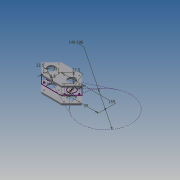
# Autodesk Inventor part: Part5
Saved by Autodesk Inventor 2013 (Build 170138000, 138)
## iProperties
Created: 2017-03-27
Part Number: Part5
Material: Generic
Document SubType Name: Modeling
Designer: employee
Density: 1 g/cm^3
Author: employee
Autodesk Inventor part; units mm, degrees
ref_plane "YZ Plane" through (0, 0, 0) normal (1, 0, 0) x (0, 1, 0)
ref_plane "XZ Plane" through (0, 0, 0) normal (0, 1, 0) x (-1, 0, 0)
ref_plane "XY Plane" through (0, 0, 0) normal (0, 0, 1) x (1, 0, 0)
sketch "Sketch1" plane through (0, 0, 0) normal (0, 0, 1) x (1, 0, 0)
  circle A0 centre (0, 0) radius 5.093 construction
  circle A1 centre (99, 0) radius 74.8028 construction
  line L0 (46.3283, 53.1146) -> (-3.5862, 3.6163) construction
  line L1 (-3.5862, -3.6163) -> (46.3283, -53.1146) construction
  circle A2 centre (-60, 0) radius 5.093 construction
  line L2 (66.2044, 67.2303) -> (-62.2329, 4.5774) construction
  line L3 (66.2044, -67.2303) -> (-62.2329, -4.5774) construction
  line L4 (-60, -29.6985) -> (-89.6985, 0) construction
  line L5 (-89.6985, 0) -> (-60, 29.6985) construction
  line L6 (-60, 29.6985) -> (-30.3015, 0) construction
  line L7 (-30.3015, 0) -> (-60, -29.6985) construction
  line L8 (-29.6985, 0) -> (0, 29.6985) construction
  line L9 (0, 29.6985) -> (29.6985, 0) construction
  line L10 (29.6985, 0) -> (0, -29.6985) construction
  line L11 (0, -29.6985) -> (-29.6985, 0) construction
  circle A3 centre (-60, 0) radius 11.25
  circle A4 centre (0, 0) radius 11.25
  line L12 (-21.9203, 0) -> (0, 21.9203) construction
  line L13 (0, 21.9203) -> (21.9203, 0) construction
  line L14 (21.9203, 0) -> (0, -21.9203) construction
  line L15 (0, -21.9203) -> (-21.9203, 0) construction
  line L16 (-60, 21.9203) -> (-38.0797, 0) construction
  line L17 (-38.0797, 0) -> (-60, -21.9203) construction
  line L18 (-60, -21.9203) -> (-81.9203, 0) construction
  line L19 (-81.9203, 0) -> (-60, 21.9203) construction
  circle A5 centre (-81.9203, 0) radius 1.75
  circle A6 centre (-60, 21.9203) radius 1.75
  circle A7 centre (-38.0797, 0) radius 1.75
  circle A8 centre (-60, -21.9203) radius 1.75
  circle A9 centre (0, -21.9203) radius 1.75
  circle A10 centre (-21.9203, 0) radius 1.75
  circle A11 centre (0, 21.9203) radius 1.75
  circle A12 centre (21.9203, 0) radius 1.75
  line L20 (-89.6985, 0) -> (-60, 29.6985)
  line L21 (-60, 29.6985) -> (0, 29.6985)
  line L22 (0, 29.6985) -> (29.6985, 0)
  line L23 (29.6985, 0) -> (0, -29.6985)
  line L24 (0, -29.6985) -> (-60, -29.6985)
  line L25 (-60, -29.6985) -> (-89.6985, 0)
  line L26 (-9.9329, 18.9203) -> (10.7782, 18.9203)
  dimension "d0" = 10.1859
  dimension "d2" = 149.6056
  dimension "d3" = 99
  dimension "d6" = 159
  dimension "d7" = 42
  dimension "d8" = 22.5
  dimension "d9" = 22.5
  dimension "d10" = 31
  dimension "d11" = 3.5
  dimension "d17" = 3
  constraints: 54 end point, 15 coincident, 13 centre point, 8 equal radius, 8 point on circle, 8 tangent, 5 parallel, 4 horizontal alignment, 2 equal length, 2 perpendicular, 1 collinear, 1 horizontal, 1 point on line, 36 other
  measures "d0" diameter of A0
  measures "d2" diameter of A1
  measures "d3" distance of A1.centre point (0, 0)
  measures "d6" distance of A1.centre A2.centre
  measures "d7" distance of L5.end L6.end
  measures "d8" diameter of A3
  measures "d9" diameter of A4
  measures "d10" distance of L18.end L16.start
  measures "d11" diameter of A5
  measures "d17" distance from line of L12.end L26
extrude "Extrusion1" add sketch "Sketch1" along normal mid plane 50
extrude "Extrusion3" cut sketch "Sketch1" along normal mid plane 40
body "Solid1"
